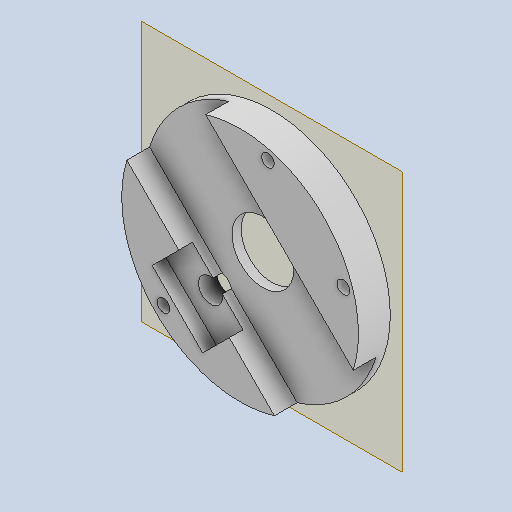
# Autodesk Inventor part: Matchboxscope_sample_v1
Saved by Autodesk Inventor 2022 (Build 260153000, 153)
## iProperties
Created: 2022-04-02
Part Number: Matchboxscope_sample_v1
Material: Generic
Document SubType Name: Modeling
Designer: Prakash Lab
Density: 1 g/cm^3
Appearance: Default
Author: Prakash Lab
Autodesk Inventor part; units mm, degrees
ref_plane "YZ Plane" through (0, 0, 0) normal (1, 0, 0) x (0, 1, 0)
ref_plane "XZ Plane" through (0, 0, 0) normal (0, 1, 0) x (-1, 0, 0)
ref_plane "XY Plane" through (0, 0, 0) normal (0, 0, 1) x (1, 0, 0)
ref_plane "Work Plane1" through (0, 0, 0) normal (0, 0, 1) x (1, 0, 0)
sketch "Sketch1" plane through (0, 0, 0) normal (0, 0, 1) x (1, 0, 0)
  circle A0 centre (0, 0) radius 25.9979 projected
  circle A1 centre (-9.4998, -11.0022) radius 2.6601 projected
  circle A2 centre (0.0001, -0.0022) radius 3.8801 projected
  circle A3 centre (0.0001, -0.0022) radius 6.7754 projected
  point P0 (0, 0)
extrude "Extrusion1" add sketch "Sketch1" along normal blind 7 contours A0
sketch "Sketch2" plane through (0, 0, 7) normal (0, 0, 1) x (1, 0, 0)
  line L0 (32.4435, -15.1193) -> (-15.1193, 32.4435)
  line L1 (-15.1193, 32.4435) -> (-32.4435, 15.1193)
  line L2 (-32.4435, 15.1193) -> (15.1193, -32.4435)
  line L3 (15.1193, -32.4435) -> (32.4435, -15.1193)
  line L4 (32.4435, -15.1193) -> (-32.4435, 15.1193) construction
  line L5 (-15.1193, 32.4435) -> (15.1193, -32.4435) construction
  line L6 (32.4435, -15.1193) -> (99.7074, -15.1193) construction
  point P0 (0, 0)
  dimension "d2" = 135
  dimension "d3" = 24.5
  constraints: 14 end point, 2 midpoint, 2 parallel, 1 equal length, 1 horizontal, 1 perpendicular
  measures "d2" angle of L6 L0
  measures "d3" distance of L1.end L0.end
extrude "Extrusion2" cut sketch "Sketch2" against normal blind 5
sketch "Sketch3" plane through (0, 0, 7) normal (0, 0, 1) x (1, 0, 0)
  line L0 (-7.7936, -20.2561) -> (-2.9652, -15.4277) projected
  line L1 (-18.7537, -9.2959) -> (-13.9253, -4.4675) projected
  line L2 (-13.5111, -3.9119) -> (-2.4095, -15.0135)
  line L3 (-2.4095, -15.0135) -> (-8.2078, -20.8117)
  line L4 (-8.2078, -20.8117) -> (-19.3094, -9.7102)
  line L5 (-19.3094, -9.7102) -> (-13.5111, -3.9119)
  line L6 (-8.9176, -8.4066) -> (-24.8767, 7.5526) projected
  line L7 (-13.4617, -3.8624) -> (-2.4095, -15.0135)
  line L8 (-2.4095, -15.0135) -> (-0.3384, -12.9607)
  line L9 (-0.3384, -12.9607) -> (-11.3905, -1.8096)
  line L10 (-11.3905, -1.8096) -> (-13.4617, -3.8624)
  line L11 (-13.4617, -3.8624) -> (-13.5111, -3.9119)
  line L12 (-8.9176, -8.4066) -> (-24.8767, 7.5526) projected
  line L13 (-13.9253, -4.4675) -> (-2.9652, -15.4277) projected
  line L14 (-7.7936, -20.2561) -> (-18.7537, -9.2959) projected
  point P0 (0, 0)
  dimension "d6" = 0.1
  constraints: 18 end point, 2 parallel, 2 perpendicular, 1 point on line
  measures "d6" distance between parallel lines of L1 L5
extrude "Extrusion3" cut sketch "Sketch3" against normal blind 3 contours L14 L1 L13 L0 | L11 L7 L2 | L2 L3 L4 L5 | L7 L10 L9 L8
sketch "Skizze4" plane through (0, 0, 7) normal (0, 0, 1) x (1, 0, 0)
  spline S0 degree 2 poles (24.1427, 2.2394) (24.731, 1.8489) (25.3785, 0.5587) (25.3785, -0.3311) knots 0 0 0 1 2 2 2 construction
  spline S1 degree 2 poles (25.3785, -0.3311) (25.3785, -1.1665) (24.7013, -2.5111) (24.1328, -2.8867) knots 0 0 0 1 2 2 2 construction
  spline S2 degree 2 poles (24.1328, -2.8867) (23.6682, -3.1784) (22.7141, -3.3761) (21.9726, -3.3761) knots 0 0 0 1 2 2 2 construction
  line L0 (21.9726, -3.3761) -> (20.5687, -3.3761) construction
  line L1 (20.5687, -3.3761) -> (20.5687, 2.7239) construction
  line L2 (20.5687, 2.7239) -> (21.9578, 2.7239) construction
  spline S3 degree 2 poles (21.9578, 2.7239) (22.8179, 2.7239) (23.7967, 2.4668) (24.1427, 2.2394) knots 0 0 0 1 2 2 2 construction
  spline S4 degree 2 poles (19.1896, -2.9312) (18.8979, -3.1982) (18.1564, -3.4849) (17.5978, -3.4849) knots 0 0 0 1 2 2 2 construction
  spline S5 degree 2 poles (17.5978, -3.4849) (16.9354, -3.4849) (16.0061, -3.2081) (15.5958, -3.0103) knots 0 0 0 1 2 2 2 construction
  line L3 (15.5958, -3.0103) -> (15.5958, -1.992) construction
  line L4 (15.5958, -1.992) -> (15.6551, -1.992) construction
  spline S6 degree 2 poles (15.6551, -1.992) (16.0555, -2.3677) (17.0689, -2.7829) (17.5385, -2.7829) knots 0 0 0 1 2 2 2 construction
  spline S7 degree 2 poles (17.5385, -2.7829) (18.2108, -2.7829) (18.8979, -2.2243) (18.8979, -1.7646) knots 0 0 0 1 2 2 2 construction
  spline S8 degree 2 poles (18.8979, -1.7646) (18.8979, -1.3988) (18.5371, -0.944) (18.1465, -0.8303) knots 0 0 0 1 2 2 2 construction
  spline S9 degree 2 poles (18.1465, -0.8303) (17.8648, -0.7513) (17.3952, -0.6425) (17.0442, -0.5535) knots 0 0 0 1 2 2 2 construction
  spline S10 degree 2 poles (17.0442, -0.5535) (16.7278, -0.4695) (16.2285, -0.2174) (16.0358, -0.0147) knots 0 0 0 1 2 2 2 construction
  spline S11 degree 2 poles (16.0358, -0.0147) (15.8479, 0.188) (15.6403, 0.7317) (15.6403, 1.0876) knots 0 0 0 1 2 2 2 construction
  spline S12 degree 2 poles (15.6403, 1.0876) (15.6403, 1.8291) (16.797, 2.8326) (17.6918, 2.8326) knots 0 0 0 1 2 2 2 construction
  spline S13 degree 2 poles (17.6918, 2.8326) (18.2059, 2.8326) (19.1154, 2.6299) (19.5059, 2.4372) knots 0 0 0 1 2 2 2 construction
  line L5 (19.5059, 2.4372) -> (19.5059, 1.4683) construction
  line L6 (19.5059, 1.4683) -> (19.4466, 1.4683) construction
  spline S14 degree 2 poles (19.4466, 1.4683) (19.155, 1.7352) (18.2454, 2.1307) (17.7461, 2.1307) knots 0 0 0 1 2 2 2 construction
  spline S15 degree 2 poles (17.7461, 2.1307) (17.1826, 2.1307) (16.4856, 1.6017) (16.4856, 1.1717) knots 0 0 0 1 2 2 2 construction
  spline S16 degree 2 poles (16.4856, 1.1717) (16.4856, 0.7861) (16.8959, 0.3264) (17.2815, 0.2226) knots 0 0 0 1 2 2 2 construction
  spline S17 degree 2 poles (17.2815, 0.2226) (17.5385, 0.1534) (18.285, -0.0246) (18.5321, -0.0987) knots 0 0 0 1 2 2 2 construction
  spline S18 degree 2 poles (18.5321, -0.0987) (19.1599, -0.2915) (19.7432, -1.0676) (19.7432, -1.6361) knots 0 0 0 1 2 2 2 construction
  spline S19 degree 2 poles (19.7432, -1.6361) (19.7432, -1.997) (19.4516, -2.689) (19.1896, -2.9312) knots 0 0 0 1 2 2 2 construction
  circle A0 centre (-9.9998, 17.4978) radius 1.3999 construction
  circle A1 centre (10.0001, 17.4979) radius 1.4 construction
  circle A2 centre (10.0001, -17.5021) radius 1.4 construction
  circle A3 centre (-9.9998, -17.5021) radius 1.4001 construction
  arc A4 (-25.1198, 6.6998) -> (-24.1417, 5.4917) centre (-24.1417, 6.4917) ccw construction
  line L7 (-24.1417, 5.4917) -> (-17.7002, 5.4917) construction
  arc A5 (-15.7002, 3.4917) -> (-17.7002, 5.4917) centre (-17.7002, 3.4917) ccw construction
  line L8 (-15.7002, 3.4917) -> (-15.7002, -4.496) construction
  arc A6 (-17.7002, -6.496) -> (-15.7002, -4.496) centre (-17.7002, -4.496) ccw construction
  line L9 (-17.7002, -6.496) -> (-23.8502, -6.496) construction
  arc A7 (-23.8502, -6.496) -> (-24.8235, -7.7254) centre (-23.8502, -7.496) ccw construction
  arc A8 (-24.8235, -7.7254) -> (-25.1198, 6.6998) centre (0, 0) ccw construction
  circle A9 centre (-9.4998, -11.0022) radius 2.6601 construction
  circle A10 centre (-16.8291, -16.0482) radius 1.4 construction
  circle A11 centre (6.1284, 23.0202) radius 1.4 construction
  circle A12 centre (22.7119, 7.1872) radius 1.4 construction
  circle A13 centre (0.0001, -0.0022) radius 6.5 construction
  point P0 (0, 0)
hole "Bohrung1" at (6.1284, 23.0202, 7) at (22.7119, 7.1872, 7) at (-16.8291, -16.0482, 7) direction (0, 0, -1) diameter 2.8 end through all
body "Solid1"
